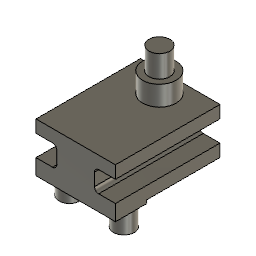
Master Slider (Autodesk Fusion 360 design; units mm, degrees)
Autodesk Fusion 360 part; units mm, degrees
sketch "Sketch1" plane through (0, 0, 0) normal (0, 0, 1) x (1, 0, 0)
  line L0 (0, 0) -> (19, 0)
  line L1 (19, 0) -> (19, 25)
  line L2 (19, 25) -> (0, 25)
  line L3 (0, 25) -> (0, 0)
  line L4 (9.5, 25) -> (9.5, 0) construction
  line L5 (0, 20) -> (19, 20) construction
  line L6 (0, 5) -> (19, 5) construction
  line L7 (5, 0) -> (5, 25) construction
  line L8 (15, 0) -> (15, 25) construction
  dimension "d1" = 19
  dimension "d2" = 25
  constraint horizontal L0
  constraint vertical L1
  constraint horizontal L2
  constraint vertical L3
  constraint coincident L0.start L3.end
  constraint midpoint L2 L4.start
  constraint midpoint L0 L4.end
  constraint coincident L3 L5.start
  constraint coincident L1 L5.end
  constraint perpendicular L1 L5
  constraint coincident L3 L6.start
  constraint coincident L1 L6.end
  constraint perpendicular L1 L6
  constraint coincident L0 L7.start
  constraint coincident L2 L7.end
  constraint perpendicular L2 L7
  constraint coincident L0 L8.start
  constraint coincident L2 L8.end
  constraint perpendicular L2 L8
  measures "d1" distance of L0.start L0.end
  measures "d2" distance of L0.start L2.end
extrude "Extrude1" add sketch "Sketch1" along normal blind 3
sketch "Sketch2" plane through (0, 0, 3) normal (0, 0, 1) x (-1, 0, 0)
  line L0 (0, -25) -> (0, 0)
  line L1 (0, 0) -> (-19, 0)
  line L2 (-19, 0) -> (-19, -25)
  line L3 (-19, -25) -> (0, -25)
  line L4 (-9.5, 0) -> (-9.5, -25) construction
  line L5 (-9.5, 0) -> (-14, 0) construction
  line L6 (-14, 0) -> (-5, 0)
  line L7 (-5, 0) -> (-5, -25)
  line L8 (-5, -25) -> (-14, -25)
  line L9 (-14, -25) -> (-14, 0)
  dimension "d5" = 4.5
  dimension "d6" = 9
  constraint midpoint L1 L4.start
  constraint midpoint L3 L4.end
  constraint perpendicular L4 L5
  constraint horizontal L6
  constraint vertical L7
  constraint horizontal L8
  constraint vertical L9
  measures "d5" distance of L4.start L5.end
  measures "d6" distance of L5.end L6.end
extrude "Extrude2" add sketch "Sketch2" along normal blind 5 contours L1 L3 L6 L7 L8 L9
fillet "Fillet1" radius 1 1 edges at (5, 12.5, 3)
fillet "Fillet2" radius 1 1 edges at (14, 12.5, 3)
sketch "Sketch3" plane through (0, 0, 8) normal (0, 0, 1) x (-1, 0, 0)
  line L0 (-14, -25) -> (-5, -25)
  line L1 (-5, -25) -> (-5, 0)
  line L2 (-5, 0) -> (-14, 0)
  line L3 (-14, 0) -> (-14, -25)
  line L4 (0, 0) -> (-19, 0)
  line L5 (-19, 0) -> (-19, -25)
  line L6 (-19, -25) -> (0, -25)
  line L7 (0, -25) -> (0, 0)
  constraint horizontal L4
  constraint vertical L5
  constraint horizontal L6
  constraint vertical L7
  constraint coincident L4.start L7.end
extrude "Extrude3" add sketch "Sketch3" along normal blind 3
fillet "Fillet3" radius 1 1 edges at (5, 12.5, 8)
fillet "Fillet4" radius 1 1 edges at (14, 12.5, 8)
sketch "Sketch4" plane through (0, 0, 0) normal (0, 0, -1) x (1, 0, 0)
  line L0 (0, 0) -> (0, -25)
  line L1 (0, -25) -> (19, -25)
  line L2 (19, -25) -> (19, 0)
  line L3 (19, 0) -> (0, 0)
  line L4 (9.5, -25) -> (9.5, 0) construction
  line L5 (9.5, -25) -> (14.5, -25) construction
  line L6 (9.5, -25) -> (4.5, -25) construction
  line L7 (14.5, -25) -> (14.5, 0) construction
  line L8 (4.5, -25) -> (4.5, 0) construction
  line L9 (9.5, -25) -> (9.5, -20) construction
  line L10 (9.5, -20) -> (14.5, -20) construction
  line L11 (10, -5) -> (14.5, -5) construction
  line L12 (9, -5) -> (4.5, -5) construction
  line L13 (9.5, -20) -> (4.5, -20) construction
  circle A0 centre (14.5, -20) radius 2.5
  circle A1 centre (4.5, -20) radius 2.5
  circle A2 centre (14.5, -5) radius 2.5
  circle A3 centre (4.5, -5) radius 2.5
  dimension "d19" = 5
  dimension "d20" = 5
  dimension "d21" = 5
  dimension "d22" = 5
  dimension "d23" = 5
  dimension "d24" = 5
  constraint midpoint L1 L4.start
  constraint midpoint L3 L4.end
  constraint coincident L1 L5.end
  constraint perpendicular L4 L6
  constraint coincident L3 L7.end
  constraint perpendicular L3 L7
  constraint coincident L3 L8.end
  constraint perpendicular L3 L8
  constraint coincident L4 L9.end
  constraint coincident L7 L10.end
  constraint perpendicular L7 L10
  constraint coincident L7 L11.end
  constraint perpendicular L7 L11
  constraint coincident L8 L12.end
  constraint perpendicular L8 L12
  constraint coincident L8 L13.end
  constraint perpendicular L8 L13
  constraint coincident L10.end A0.centre
  constraint coincident L13.end A1.centre
  constraint coincident L11.end A2.centre
  constraint coincident L12.end A3.centre
  measures "d19" distance of L4.start L5.end
  measures "d20" distance of L4.start L6.end
  measures "d21" diameter of A0
  measures "d22" diameter of A1
  measures "d23" diameter of A2
  measures "d24" diameter of A3
extrude "Extrude4" add sketch "Sketch4" along normal blind 4 contours A0 | A1 | A2 | A3
sketch "Sketch5" plane through (0, 0, 11) normal (0, 0, 1) x (-1, 0, 0)
  line L0 (0, -25) -> (0, 0)
  line L1 (0, 0) -> (-19, 0)
  line L2 (-19, 0) -> (-19, -25)
  line L3 (-19, -25) -> (0, -25)
  line L4 (-9.5, 0) -> (-9.5, -5) construction
  circle A0 centre (-9.5, -5) radius 2.5
  constraint midpoint L1 L4.start
  constraint perpendicular L1 L4
  constraint coincident L4.end A0.centre
extrude "Extrude5" add sketch "Sketch5" along normal blind 4 contours A0
sketch "Sketch6" plane through (0, 0, 11) normal (0, 0, 1) x (-1, 0, 0)
  circle A0 centre (-9.5, -5) radius 2.5
  line L0 (0, -25) -> (0, 0)
  line L1 (0, 0) -> (-19, 0)
  line L2 (-19, 0) -> (-19, -25)
  line L3 (-19, -25) -> (0, -25)
  line L4 (-9.5, -5) -> (-9.5, 0) construction
  line L5 (-9.5, -25) -> (-9.5, -20) construction
  circle A1 centre (-9.5, -20) radius 2.5
  dimension "d29" = 5
  constraint coincident A0.centre L4.start
  constraint midpoint L1 L4.end
  constraint midpoint L3 L5.start
  constraint perpendicular L3 L5
  constraint coincident L5.end A1.centre
  measures "d29" diameter of A1
extrude "Extrude6" add sketch "Sketch6" along normal blind 10 contours A1
extrude "Extrude7" cut 1 faces at (9.5732, 5.685, 15) along direction (0, 0, -1) blind 4
sketch "Sketch7" plane through (0, 0, 11) normal (0, 0, 1) x (-1, 0, 0)
  circle A0 centre (-9.5, -20) radius 2.5
  line L0 (0, -25) -> (0, 0)
  line L1 (0, 0) -> (-19, 0)
  line L2 (-19, 0) -> (-19, -25)
  line L3 (-19, -25) -> (0, -25)
  circle A1 centre (-9.5, -20) radius 5
  constraint concentric A0 A1
  constraint tangent L3 A1
extrude "Extrude8" add sketch "Sketch7" along normal blind 5 contours A1
sketch "Sketch8" plane through (0, 0, 16) normal (0, 0, 1) x (-1, 0, 0)
  circle A0 centre (-9.5, -20) radius 2.5
  circle A1 centre (-9.5, -20) radius 5
  circle A2 centre (-9.5, -20) radius 4
  dimension "d36" = 8
  constraint concentric A0 A2
  measures "d36" diameter of A2
extrude "Extrude9" cut sketch "Sketch8" against normal blind 5 contours A1
extrude "Extrude10" add 1 faces at (6.0149, 20.1987, 16) along direction (0, 0, 1) blind 4.727
extrude "Extrude11" add 1 faces at (9.4377, 21.5541, 21) along direction (0, 0, 1) blind 5
extrude "Extrude12" cut 1 faces at (6.0149, 20.1987, 20.727) along direction (0, 0, -1) blind 5
extrude "Extrude13" cut 1 faces at (9.4377, 21.5541, 26) along direction (0, 0, -1) blind 5
extrude "Extrude14" cut 2 faces at (5.2162, 19.1607, -4) (15.2256, 20.7151, -4) along direction (0, 0, 1) blind 4
extrude "Extrude15" cut 2 faces at (15.2963, 5.4775, -4) (4.4377, 4.2795, -4) along direction (0, 0, 1) blind 4
sketch "Sketch9" plane through (0, 0, 0) normal (0, 0, -1) x (1, 0, 0)
  line L0 (0, 0) -> (0, -25)
  line L1 (0, -25) -> (19, -25)
  line L2 (19, -25) -> (19, 0)
  line L3 (19, 0) -> (0, 0)
  line L4 (9.5, 0) -> (9.5, -5) construction
  line L5 (9.5, -5) -> (16, -5) construction
  line L6 (9.5, -5) -> (3, -5) construction
  circle A0 centre (16, -5) radius 2.5
  circle A1 centre (3, -5) radius 2.5
  dimension "d51" = 5
  dimension "d52" = 6.5
  dimension "d53" = 6.5
  dimension "d54" = 5
  dimension "d55" = 5
  constraint midpoint L3 L4.start
  constraint perpendicular L1 L4
  constraint perpendicular L2 L5
  constraint perpendicular L4 L6
  constraint coincident L5.end A0.centre
  constraint coincident L6.end A1.centre
  measures "d51" distance of L4.start L4.end
  measures "d52" distance of L4.end L5.end
  measures "d53" distance of L4.end L6.end
  measures "d54" diameter of A0
  measures "d55" diameter of A1
extrude "Extrude16" add sketch "Sketch9" along normal blind 5 contours A0 | A1
extrude "Extrude17" add 2 faces at (3.2442, 4.3779, -5) (16.0752, 4.7003, -5) along direction (0, 0, -1) blind 0.773
sketch "Sketch10" plane through (0, 0, 0) normal (0, 0, -1) x (1, 0, 0)
  circle A0 centre (3, -5) radius 2.5
  circle A1 centre (16, -5) radius 2.5
  line L0 (0, 0) -> (0, -25)
  line L1 (0, -25) -> (19, -25)
  line L2 (19, -25) -> (19, 0)
  line L3 (19, 0) -> (0, 0)
  line L4 (16, -5) -> (19, -5) construction
  line L5 (19, -5) -> (19, -7.5) construction
  line L6 (19, -7.5) -> (0, -7.5)
  line L7 (0, -7.5) -> (0, 0)
  line L8 (0, 0) -> (19, 0)
  line L9 (19, 0) -> (19, -7.5)
  dimension "d60" = 2.5
  constraint coincident A1.centre L4.start
  constraint coincident L2 L4.end
  constraint perpendicular L2 L4
  constraint perpendicular L4 L5
  constraint horizontal L6
  constraint vertical L7
  constraint horizontal L8
  constraint vertical L9
  constraint coincident L0.start L3.end
  measures "d60" distance of L4.end L5.end
extrude "Extrude18" add sketch "Sketch10" along normal blind 0.773 contours L0 L2 L3 L6 L7 L8 L9
